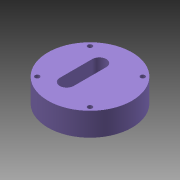
# Autodesk Inventor part: Arm Plate
Saved by Autodesk Inventor 2015 (Build 190159000, 159)
## iProperties
Created: 2015-12-04
Part Number: Arm Plate
Material: Generic
Document SubType Name: Modeling
Designer: Eli
Density: 1 g/cm^3
Appearance: Default
Author: Eli
Autodesk Inventor part; units mm, degrees
ref_plane "YZ Plane" through (0, 0, 0) normal (1, 0, 0) x (0, 1, 0)
ref_plane "XZ Plane" through (0, 0, 0) normal (0, 1, 0) x (-1, 0, 0)
ref_plane "XY Plane" through (0, 0, 0) normal (0, 0, 1) x (1, 0, 0)
sketch "Sketch1" plane through (0, 0, 0) normal (0, 0, 1) x (1, 0, 0)
  circle A0 centre (0, 0) radius 45
  line L0 (-7.5, 25) -> (-7.5, 25)
  line L1 (-15, 17.5) -> (-15, -17.5)
  line L2 (-7.5, -25) -> (-7.5, -25)
  line L3 (0, -17.5) -> (0, 17.5)
  arc A1 (-7.5, 25) -> (-15, 17.5) centre (-7.5, 17.5) ccw
  arc A2 (-15, -17.5) -> (-7.5, -25) centre (-7.5, -17.5) ccw
  arc A3 (-7.5, -25) -> (0, -17.5) centre (-7.5, -17.5) ccw
  arc A4 (0, 17.5) -> (-7.5, 25) centre (-7.5, 17.5) ccw
  point P0 (-15, -25)
  point P1 (-15, 25)
  point P2 (0, -25)
  dimension "d0" = 90
  dimension "d1" = 15
  dimension "d2" = 50
  dimension "d3" = 7.5
  dimension "d4" = 25
  dimension "d5" = 0
  constraints: 8 end point, 8 point on circle, 8 tangent, 6 point on line, 5 centre point, 3 equal radius, 2 parallel, 1 coincident, 1 horizontal, 1 perpendicular
  measures "d0" diameter of A0
  measures "d1" distance of point (0, -25) point (-15, -25)
  measures "d2" distance of point (-15, -25) point (-15, 25)
  measures "d3" radius of A1
  measures "d4" distance from line of point (0, 0) L0
  measures "d5" distance from line of point (0, 0) L3
extrude "Extrusion1" add sketch "Sketch1" along normal blind 25
sketch "Sketch2" plane through (0, 0, 25) normal (0, 0, 1) x (1, 0, 0)
  line L0 (0, 0) -> (-28.2843, 28.2843)
  line L1 (0, 0) -> (40, 0) construction
  circle A0 centre (-28.2843, 28.2843) radius 2.5
  dimension "d8" = 40
  dimension "d9" = 135
  dimension "d10" = 5
  constraints: 4 end point, 1 centre point, 1 coincident, 1 equal length, 1 horizontal
  measures "d8" distance of L0.start L0.end
  measures "d9" angle of L1 L0
  measures "d10" diameter of A0
extrude "Extrusion2" cut sketch "Sketch2" against normal blind 23
pattern_circular "Circular Pattern1" count 4 over 360 about axis through (0, 0, 0) along (0, 0, 1) of "Extrusion2"
sketch "Sketch3" plane through (-28.2843, 28.2843, 2) normal (0, 0, 1) x (1, 0, 0)
  circle A0 centre (0, 0) radius 1.25
  point P0 (28.2843, -28.2843)
  dimension "d16" = 2.5
  constraints: 1 centre point
  measures "d16" diameter of A0
extrude "Extrusion3" cut sketch "Sketch3" against normal blind 3
pattern_circular "Circular Pattern2" count 4 over 360 about axis through (0, 0, 0) along (0, 0, 1) of "Extrusion3"
body "Solid1"
